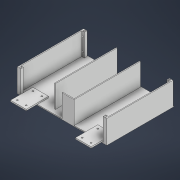
# Autodesk Inventor part: Grundplatte_hinten
Saved by Autodesk Inventor 2021 (Build 250183000, 183)
## iProperties
Created: 2021-01-26
Part Number: Grundplatte_hinten
Material: Generisch
Document SubType Name: Modeling
Designer: Ctroi
Density: 1 g/cm^3
Appearance: Vorgabe
Author: Ctroi
## iProperties of the stored document _3D-Druck.ipt
Created: 2021-01-26
Part Number: _3D-Druck
Material: Generisch
Document SubType Name: Modeling
Designer: Ctroi
Density: 1 g/cm^3
Appearance: Vorgabe
Author: Ctroi
Autodesk Inventor part; units mm, degrees
ref_plane "YZ Plane" through (0, 0, 0) normal (1, 0, 0) x (0, 1, 0)
ref_plane "XZ Plane" through (0, 0, 0) normal (0, 1, 0) x (-1, 0, 0)
ref_plane "XY Plane" through (0, 0, 0) normal (0, 0, 1) x (1, 0, 0)
sketch "Skizze1" plane through (0, 0, 0) normal (0, 1, 0) x (-1, 0, 0)
  line L0 (-100, -75) -> (100, -75)
  line L1 (100, -75) -> (100, 75)
  line L2 (100, 75) -> (-100, 75)
  line L3 (-100, 75) -> (-100, -75)
  line L4 (0, -105) -> (0, 105) projected
  line L5 (-140, 0) -> (140, 0) projected
  point P0 (0, 0)
  dimension "d0" = 200
  dimension "d1" = 150
  constraints: 8 end point, 2 parallel, 1 horizontal, 1 perpendicular, 2 other
  measures "d0" distance of L1.end L2.end
  measures "d1" distance of L0.end L1.end
extrude "Extrusion1" add sketch "Skizze1" along normal blind 2
sketch "Skizze2" plane through (0, 2, 0) normal (0, 1, 0) x (1, 0, 0)
  line L0 (-90, -100) -> (-55, -100)
  line L1 (-55, -100) -> (-55, -50)
  line L2 (-55, -50) -> (-90, -50)
  line L3 (-90, -50) -> (-90, -100)
  line L4 (-100, -75) -> (100, -75) projected
  line L5 (-100, 75) -> (-100, -75) projected
  line L6 (0, 110) -> (0, -135) projected
  line L7 (90, -100) -> (55, -100)
  line L8 (55, -100) -> (55, -50)
  line L9 (55, -50) -> (90, -50)
  line L10 (90, -50) -> (90, -100)
  point P0 (0, 0)
  dimension "d4" = 35
  dimension "d5" = 50
  dimension "d6" = 10
  constraints: 16 end point, 4 symmetric about line, 2 parallel, 1 horizontal, 1 perpendicular, 1 other
  measures "d4" distance of L2.end L1.end
  measures "d5" distance of L1.end L0.end
  measures "d6" distance between parallel lines of L5 L3
extrude "Extrusion2" add sketch "Skizze2" along normal blind 3
sketch "Skizze3" plane through (0, 5, 0) normal (0, 1, 0) x (1, 0, 0)
  circle A0 centre (-82.5, -92.5) radius 1.6
  circle A1 centre (-62.5, -92.5) radius 1.6
  circle A2 centre (-82.5, -57.5) radius 1.6
  circle A3 centre (-62.5, -57.5) radius 1.6
  line L0 (-55, -100) -> (-55, -50) projected
  line L1 (-90, -50) -> (-90, -100) projected
  line L2 (-90, -100) -> (-55, -100) projected
  line L3 (-55, -50) -> (-90, -50) projected
  line L4 (0, 110) -> (0, -135) projected
  circle A4 centre (82.5, -92.5) radius 1.6
  circle A5 centre (62.5, -92.5) radius 1.6
  circle A6 centre (82.5, -57.5) radius 1.6
  circle A7 centre (62.5, -57.5) radius 1.6
  point P0 (0, 0)
  dimension "d9" = 3.2
  dimension "d10" = 3.2
  dimension "d11" = 3.2
  dimension "d12" = 3.2
  dimension "d13" = 7.5
  dimension "d14" = 7.5
  dimension "d15" = 7.5
  dimension "d16" = 7.5
  dimension "d17" = 7.5
  dimension "d18" = 7.5
  dimension "d19" = 7.5
  dimension "d20" = 7.5
  constraints: 8 centre point, 4 symmetric about line, 4 other
  measures "d9" diameter of A0
  measures "d10" diameter of A1
  measures "d11" diameter of A2
  measures "d12" diameter of A3
  measures "d13" distance from line of L0 A3.centre
  measures "d14" distance from line of L1 A2.centre
  measures "d15" distance from line of L1 A0.centre
  measures "d16" distance from line of L0 A1.centre
  measures "d17" distance from line of L2 A1.centre
  measures "d18" distance from line of L2 A0.centre
  measures "d19" distance from line of L3 A2.centre
  measures "d20" distance from line of L3 A3.centre
extrude "Extrusion3" cut sketch "Skizze3" against normal up to surface (5 mm away) contours A0 | A1 | A2 | A3 | A4 | A5 | A6 | A7
sketch "Skizze4" plane through (0, 2, 0) normal (0, 1, 0) x (1, 0, 0)
  line L0 (100, 75) -> (-100, 75) projected
  line L1 (-27.5, 75) -> (27, 75)
  line L2 (27, 73) -> (27, -75)
  line L3 (27, -75) -> (-28, -75)
  line L4 (-27, -64.901) -> (-27, 73)
  line L5 (0, 105) -> (0, -105) projected
  line L6 (25, 73) -> (25, -73)
  line L7 (25, -73) -> (-16, -73)
  line L8 (-25, -64.901) -> (-25, 73)
  line L9 (-55, -75) -> (55, -75) projected
  line L10 (-16, -73) -> (-16, -75)
  line L11 (-16, -75) -> (-6, -75)
  line L12 (-100, 75) -> (-100, -75) projected
  line L13 (-27, -64.901) -> (-25, -64.901)
  line L14 (27, 73) -> (25, 73)
  line L15 (-25, 73) -> (-27, 73)
  line L16 (90, -75) -> (100, -75) projected
  line L17 (100, -75) -> (98, -75)
  line L18 (98, -75) -> (98, 73)
  line L19 (98, 73) -> (100, 73)
  line L20 (100, 73) -> (100, -75)
  line L21 (-100, -75) -> (-90, -75) projected
  line L22 (-100, -75) -> (-98, -75)
  line L23 (-98, -75) -> (-98, 73)
  line L24 (-98, 73) -> (-100, 73)
  line L25 (-100, 73) -> (-100, -75)
  line L26 (98, 73) -> (92, 73)
  line L27 (92, 73) -> (92, 67)
  line L28 (92, 67) -> (98, 67)
  line L29 (98, 67) -> (98, 73)
  line L30 (-98, 73) -> (-92, 73)
  line L31 (-92, 73) -> (-92, 67)
  line L32 (-92, 67) -> (-98, 67)
  line L33 (-98, 67) -> (-98, 73)
  line L34 (98, -75) -> (92, -75)
  line L35 (92, -75) -> (92, -69)
  line L36 (92, -69) -> (98, -69)
  line L37 (98, -69) -> (98, -75)
  line L38 (-98, -75) -> (-92, -75)
  line L39 (-92, -75) -> (-92, -69)
  line L40 (-92, -69) -> (-98, -69)
  line L41 (-98, -69) -> (-98, -75)
  point P0 (0, 0)
  point P1 (-25.5, 75)
  point P2 (0, -73)
  point P3 (0, -75)
  point P4 (27.5, 75)
  point P5 (-25.5, -75)
  point P6 (-16, -75)
  point P7 (-100, 73)
  point P8 (-98, -75)
  point P9 (-98, 67)
  point P10 (98, 67)
  point P11 (98, -69)
  point P12 (92, -75)
  dimension "d23" = 55
  dimension "d24" = 150
  dimension "d25" = 2
  dimension "d26" = 10
  dimension "d27" = 2
  dimension "d29" = 43
  dimension "d30" = 2
  dimension "d35" = 10.099
  dimension "d36" = 2
  dimension "d37" = 2
  dimension "d38" = 2
  dimension "d39" = 2
  dimension "d40" = 148
  dimension "d41" = 2
  dimension "d42" = 6
  dimension "d43" = 6
  dimension "d44" = 6
  dimension "d45" = 6
  dimension "d66" = 6
  dimension "d67" = 6
  dimension "d68" = 6
  dimension "d69" = 6
  dimension "d78" = 25
  dimension "d79" = 2
  constraints: 72 end point, 15 parallel, 9 perpendicular, 8 horizontal, 4 point on line, 1 other
  measures "d23" distance of L2.end L3.end
  measures "d24" distance of L1.end L2.end
  measures "d25" distance between parallel lines of L4 L8
  measures "d26" distance of L11.end L10.end
  measures "d27" distance between parallel lines of L3 L7
  measures "d29" distance between parallel lines of L2 L10
  measures "d30" distance between parallel lines of L2 L6
  measures "d35" distance between parallel lines of L9 L13
  measures "d36" distance between parallel lines of L0 L14
  measures "d37" distance between parallel lines of L0 L15
  measures "d38" distance of L18.end L19.end
  measures "d39" distance of L24.end L23.end
  measures "d40" distance of L23.end L22.end
  measures "d41" distance between parallel lines of L0 L19
  measures "d42" distance of L28.end L27.end
  measures "d43" distance of L27.end L26.end
  measures "d44" distance of L31.end L32.end
  measures "d45" distance of L30.end L31.end
  measures "d66" distance of L35.end L36.end
  measures "d67" distance of L34.end L35.end
  measures "d68" distance of L40.end L39.end
  measures "d69" distance of L39.end L38.end
  measures "d78" distance between parallel lines of L5 L8
  measures "d79" distance between parallel lines of L9 L7
extrude "Extrusion7" add sketch "Skizze4" along normal blind 50 contours L2 L3 L5 L7 L6 L14 | L4 L15 L8 L13 | L24 L23 L21 L12 | L30 L31 L32 L23 | L23 L40 L39 L21 | L35 L36 L18 L16 | L18 L19 L20 L16 | L28 L27 L26 L18
sketch "Skizze7" plane through (100, 2, -73) normal (0, 0, -1) x (-1, 0, 0)
  circle A0 centre (4, 40) radius 2
  circle A1 centre (4, 10) radius 2
  line L0 (0, 0) -> (200, 0) projected
  line L1 (8, 0) -> (8, 50) projected
  line L2 (0, 50) -> (8, 50) projected
  circle A2 centre (196, 10) radius 2
  line L3 (192, 0) -> (192, 50) projected
  circle A3 centre (196, 40) radius 2
  line L4 (192, 50) -> (200, 50) projected
  point P0 (100, -2)
  dimension "d82" = 4
  dimension "d83" = 4
  dimension "d84" = 10
  dimension "d85" = 4
  dimension "d86" = 4
  dimension "d87" = 10
  dimension "d88" = 4
  dimension "d89" = 4
  dimension "d90" = 10
  dimension "d91" = 4
  dimension "d92" = 10
  dimension "d93" = 4
  constraints: 4 centre point
  measures "d82" diameter of A0
  measures "d83" diameter of A1
  measures "d84" distance from line of L0 A1.centre
  measures "d85" distance from line of L1 A1.centre
  measures "d86" distance from line of L1 A0.centre
  measures "d87" distance from line of L2 A0.centre
  measures "d88" diameter of A2
  measures "d89" distance from line of L3 A2.centre
  measures "d90" distance from line of L0 A2.centre
  measures "d91" diameter of A3
  measures "d92" distance from line of L4 A3.centre
  measures "d93" distance from line of L3 A3.centre
extrude "Extrusion8" cut sketch "Skizze7" against normal up to surface (6 mm away)
sketch "Skizze8" plane through (0, 52, 0) normal (0, 1, 0) x (1, 0, 0)
  circle A0 centre (95, 70) radius 2
  line L0 (100, 73) -> (92, 73) projected
  line L1 (92, 73) -> (92, 67) projected
  circle A1 centre (-95, 70) radius 2
  line L2 (-92, 73) -> (-100, 73) projected
  line L3 (-92, 67) -> (-92, 73) projected
  circle A2 centre (-95, -72) radius 2
  line L4 (-92, -69) -> (-98, -69) projected
  line L5 (-92, -75) -> (-92, -69) projected
  circle A3 centre (95, -72) radius 2
  line L6 (98, -69) -> (92, -69) projected
  line L7 (92, -69) -> (92, -75) projected
  point P0 (0, 0)
  dimension "d96" = 4
  dimension "d97" = 3
  dimension "d98" = 3
  dimension "d99" = 4
  dimension "d100" = 3
  dimension "d101" = 3
  dimension "d102" = 4
  dimension "d103" = 3
  dimension "d104" = 3
  dimension "d105" = 4
  dimension "d106" = 3
  dimension "d107" = 3
  constraints: 4 centre point
  measures "d96" diameter of A0
  measures "d97" distance from line of L0 A0.centre
  measures "d98" distance from line of L1 A0.centre
  measures "d99" diameter of A1
  measures "d100" distance from line of L2 A1.centre
  measures "d101" distance from line of L3 A1.centre
  measures "d102" diameter of A2
  measures "d103" distance from line of L4 A2.centre
  measures "d104" distance from line of L5 A2.centre
  measures "d105" diameter of A3
  measures "d106" distance from line of L6 A3.centre
  measures "d107" distance from line of L7 A3.centre
extrude "Extrusion9" cut sketch "Skizze8" against normal blind 5
